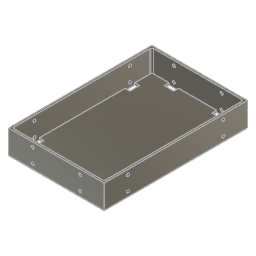
Arm Unit Bottom Case v1 (Autodesk Fusion 360 design; units mm, degrees)
Autodesk Fusion 360 part; units mm, degrees
sketch "Sketch1" plane through (0, 0, 0) normal (0, 0, 1) x (1, 0, 0) in component "case"
  line L0 (50, -75) -> (-50, -75)
  line L1 (-50, -75) -> (-50, 75)
  line L2 (-50, 75) -> (50, 75)
  line L3 (50, 75) -> (50, -75)
  line L4 (50, -75) -> (-50, 75) construction
  line L5 (-50, -75) -> (50, 75) construction
  dimension "d1" = 100
  dimension "d2" = 150
  constraint horizontal L0
  constraint perpendicular L0 L1
  constraint parallel L0 L2
  constraint parallel L1 L3
  constraint coincident L4 origin
  constraint coincident L5 origin
  measures "d1" distance of L1.end L2.end
  measures "d2" distance of L0.end L1.end
extrude "Extrude1" add sketch "Sketch1" along normal blind 25 in component "case"
sketch "Sketch1 (2)" plane through (0, 0, 25) normal (0, 0, 1) x (-1, 0, 0)
  line L0 (-50, -75) -> (50, -75)
  line L1 (50, -75) -> (50, 75)
  line L2 (50, 75) -> (-50, 75)
  line L3 (-50, 75) -> (-50, -75)
  line L4 (48, -73) -> (48, 73)
  line L5 (48, 73) -> (-48, 73)
  line L6 (-48, 73) -> (-48, -73)
  line L7 (-48, -73) -> (48, -73)
  dimension "d5" = -2
extrude "Extrude2" cut sketch "Sketch1 (2)" against normal blind 23 contours L4 L5 L6 L7 in component "case"
fillet "Fillet1" radius 2 4 edges at (48, -73, 13.5) (-48, -73, 13.5) (48, 73, 13.5) (-48, 73, 13.5) in component "case"
sketch "Sketch3" plane through (-50, 0, 0) normal (-1, 0, 0) x (0, -1, 0)
  line L0 (-75, 0) -> (75, 0)
  line L1 (75, 0) -> (75, 25)
  line L2 (75, 25) -> (-75, 25)
  line L3 (-75, 25) -> (-75, 0)
  circle A0 centre (-50, 20) radius 1.5
  dimension "d10" = 3
  measures "d10" diameter of A0
sketch "Sketch2" plane through (50, 0, 0) normal (1, 0, 0) x (0, 1, 0)
  line L0 (-75, 0) -> (75, 0)
  line L1 (75, 0) -> (75, 25)
  line L2 (75, 25) -> (-75, 25)
  line L3 (-75, 25) -> (-75, 0)
  circle A0 centre (-50, 20) radius 1.5
  dimension "d27" = 3
  measures "d27" diameter of A0
extrude "Extrude7" cut sketch "Sketch2" against normal blind 2 contours A0 in component "case"
extrude "Extrude3" cut sketch "Sketch3" against normal blind 2 contours A0 in component "case"
sketch "Sketch5" plane through (-50, 0, 0) normal (-1, 0, 0) x (0, -1, 0)
  circle A0 centre (-50, 20) radius 1.5
  line L0 (-75, 0) -> (75, 0)
  line L1 (75, 0) -> (75, 25)
  line L2 (75, 25) -> (-75, 25)
  line L3 (-75, 25) -> (-75, 0)
  circle A1 centre (-50, 5) radius 1.5
  dimension "d18" = 3
  measures "d18" diameter of A1
extrude "Extrude4" cut sketch "Sketch5" against normal blind 2 contours A1 in component "case"
sketch "Sketch6" plane through (-50, 0, 0) normal (-1, 0, 0) x (0, -1, 0)
  circle A0 centre (-50, 5) radius 1.5
  circle A1 centre (-50, 20) radius 1.5
  line L0 (-75, 0) -> (75, 0)
  line L1 (75, 0) -> (75, 25)
  line L2 (75, 25) -> (-75, 25)
  line L3 (-75, 25) -> (-75, 0)
  circle A2 centre (50, 5) radius 1.5
  dimension "d21" = 3
  measures "d21" diameter of A2
extrude "Extrude5" cut sketch "Sketch6" against normal blind 2 contours A2 in component "case"
sketch "Sketch7" plane through (-50, 0, 0) normal (-1, 0, 0) x (0, -1, 0)
  circle A0 centre (50, 5) radius 1.5
  circle A1 centre (-50, 5) radius 1.5
  circle A2 centre (-50, 20) radius 1.5
  line L0 (-75, 0) -> (75, 0)
  line L1 (75, 0) -> (75, 25)
  line L2 (75, 25) -> (-75, 25)
  line L3 (-75, 25) -> (-75, 0)
  circle A3 centre (50, 20) radius 1.5
  dimension "d24" = 3
  measures "d24" diameter of A3
extrude "Extrude6" cut sketch "Sketch7" against normal blind 2 contours A3 in component "case"
sketch "Sketch8" plane through (50, 0, 0) normal (1, 0, 0) x (0, 1, 0)
  circle A0 centre (-50, 20) radius 1.5
  line L0 (-75, 0) -> (75, 0)
  line L1 (75, 0) -> (75, 25)
  line L2 (75, 25) -> (-75, 25)
  line L3 (-75, 25) -> (-75, 0)
  circle A1 centre (-50, 5) radius 1.5
  dimension "d30" = 3
  measures "d30" diameter of A1
extrude "Extrude8" cut sketch "Sketch8" against normal blind 2 contours A1 in component "case"
sketch "Sketch9" plane through (50, 0, 0) normal (1, 0, 0) x (0, 1, 0)
  circle A0 centre (-50, 5) radius 1.5
  circle A1 centre (-50, 20) radius 1.5
  line L0 (-75, 0) -> (75, 0)
  line L1 (75, 0) -> (75, 25)
  line L2 (75, 25) -> (-75, 25)
  line L3 (-75, 25) -> (-75, 0)
  circle A2 centre (50, 20) radius 1.5
  dimension "d33" = 3
  measures "d33" diameter of A2
extrude "Extrude9" cut sketch "Sketch9" against normal blind 2 contours A2 in component "case"
sketch "Sketch10" plane through (50, 0, 0) normal (1, 0, 0) x (0, 1, 0)
  circle A0 centre (50, 20) radius 1.5
  circle A1 centre (-50, 5) radius 1.5
  circle A2 centre (-50, 20) radius 1.5
  line L0 (-75, 0) -> (75, 0)
  line L1 (75, 0) -> (75, 25)
  line L2 (75, 25) -> (-75, 25)
  line L3 (-75, 25) -> (-75, 0)
  circle A3 centre (50, 5) radius 1.5
  dimension "d36" = 3
  measures "d36" diameter of A3
extrude "Extrude10" cut sketch "Sketch10" against normal blind 2 contours A3 in component "case"
sketch "Sketch11" plane through (0, 75, 0) normal (0, 1, 0) x (-1, 0, 0)
  line L0 (-50, 0) -> (50, 0)
  line L1 (50, 0) -> (50, 25)
  line L2 (50, 25) -> (-50, 25)
  line L3 (-50, 25) -> (-50, 0)
  circle A0 centre (-25, 20) radius 1.5
  dimension "d39" = 3
  measures "d39" diameter of A0
extrude "Extrude11" cut sketch "Sketch11" against normal blind 2 contours A0 in component "case"
sketch "Sketch12" plane through (0, 75, 0) normal (0, 1, 0) x (-1, 0, 0)
  circle A0 centre (-25, 20) radius 1.5
  line L0 (-50, 0) -> (50, 0)
  line L1 (50, 0) -> (50, 25)
  line L2 (50, 25) -> (-50, 25)
  line L3 (-50, 25) -> (-50, 0)
  circle A1 centre (-25, 5) radius 1.5
  dimension "d42" = 3
  measures "d42" diameter of A1
extrude "Extrude12" cut sketch "Sketch12" against normal blind 2 contours A1 in component "case"
sketch "Sketch13" plane through (0, 75, 0) normal (0, 1, 0) x (-1, 0, 0)
  circle A0 centre (-25, 5) radius 1.5
  circle A1 centre (-25, 20) radius 1.5
  line L0 (-50, 0) -> (50, 0)
  line L1 (50, 0) -> (50, 25)
  line L2 (50, 25) -> (-50, 25)
  line L3 (-50, 25) -> (-50, 0)
  circle A2 centre (25, 5) radius 1.5
  dimension "d45" = 3
  measures "d45" diameter of A2
extrude "Extrude13" cut sketch "Sketch13" against normal blind 2 contours A2 in component "case"
sketch "Sketch14" plane through (0, 75, 0) normal (0, 1, 0) x (-1, 0, 0)
  circle A0 centre (25, 5) radius 1.5
  circle A1 centre (-25, 5) radius 1.5
  circle A2 centre (-25, 20) radius 1.5
  line L0 (-50, 0) -> (50, 0)
  line L1 (50, 0) -> (50, 25)
  line L2 (50, 25) -> (-50, 25)
  line L3 (-50, 25) -> (-50, 0)
  circle A3 centre (25, 20) radius 1.5
  dimension "d48" = 3
  measures "d48" diameter of A3
extrude "Extrude14" cut sketch "Sketch14" against normal blind 2 contours A3 in component "case"
sketch "Sketch15" plane through (0, -75, 0) normal (0, -1, 0) x (1, 0, 0)
  line L0 (-50, 0) -> (50, 0)
  line L1 (50, 0) -> (50, 25)
  line L2 (50, 25) -> (-50, 25)
  line L3 (-50, 25) -> (-50, 0)
  circle A0 centre (-25, 20) radius 1.5
  dimension "d51" = 3
  measures "d51" diameter of A0
extrude "Extrude15" cut sketch "Sketch15" against normal blind 2 contours A0 in component "case"
sketch "Sketch16" plane through (0, -75, 0) normal (0, -1, 0) x (1, 0, 0)
  circle A0 centre (-25, 20) radius 1.5
  line L0 (-50, 0) -> (50, 0)
  line L1 (50, 0) -> (50, 25)
  line L2 (50, 25) -> (-50, 25)
  line L3 (-50, 25) -> (-50, 0)
  circle A1 centre (-25, 5) radius 1.5
  dimension "d54" = 3
  measures "d54" diameter of A1
extrude "Extrude16" cut sketch "Sketch16" against normal blind 2 contours A1 in component "case"
sketch "Sketch17" plane through (0, -75, 0) normal (0, -1, 0) x (1, 0, 0)
  circle A0 centre (-25, 5) radius 1.5
  circle A1 centre (-25, 20) radius 1.5
  line L0 (-50, 0) -> (50, 0)
  line L1 (50, 0) -> (50, 25)
  line L2 (50, 25) -> (-50, 25)
  line L3 (-50, 25) -> (-50, 0)
  circle A2 centre (25, 5) radius 1.5
  dimension "d57" = 3
  measures "d57" diameter of A2
extrude "Extrude17" cut sketch "Sketch17" against normal blind 2 contours A2 in component "case"
sketch "Sketch18" plane through (0, -75, 0) normal (0, -1, 0) x (1, 0, 0)
  circle A0 centre (25, 5) radius 1.5
  circle A1 centre (-25, 5) radius 1.5
  circle A2 centre (-25, 20) radius 1.5
  line L0 (-50, 0) -> (50, 0)
  line L1 (50, 0) -> (50, 25)
  line L2 (50, 25) -> (-50, 25)
  line L3 (-50, 25) -> (-50, 0)
  circle A3 centre (25, 20) radius 1.5
  dimension "d60" = 3
  measures "d60" diameter of A3
extrude "Extrude18" cut sketch "Sketch18" against normal blind 2 contours A3 in component "case"
sketch "Sketch20" plane through (0, 0, 2) normal (0, 0, 1) x (-1, 0, 0)
  arc A0 (46, -73) -> (48, -71) centre (46, -71) ccw
  line L0 (48, -71) -> (48, 71)
  arc A1 (48, 71) -> (46, 73) centre (46, 71) ccw
  line L1 (46, 73) -> (-46, 73)
  arc A2 (-46, 73) -> (-48, 71) centre (-46, 71) ccw
  line L2 (-48, 71) -> (-48, -71)
  arc A3 (-48, -71) -> (-46, -73) centre (-46, -71) ccw
  line L3 (-46, -73) -> (46, -73)
  line L4 (-48, -45) -> (-43, -45)
  line L5 (-43, -45) -> (-43, -55)
  line L6 (-43, -55) -> (-48, -55)
  line L7 (-48, -55) -> (-48, -45)
  dimension "d65" = 5
  dimension "d66" = 10
  constraint horizontal L4
  constraint vertical L5
  constraint horizontal L6
  constraint vertical L7
  measures "d65" distance of L4.start L4.end
  measures "d66" distance of L4.start L6.end
extrude "Extrude19" cut sketch "Sketch20" against normal blind 2 contours L2 L4 L5 L6 L7 in component "case"
sketch "Sketch21" plane through (0, 0, 2) normal (0, 0, 1) x (-1, 0, 0)
  line L0 (-43, -55) -> (-48, -55)
  line L1 (-48, -55) -> (-48, -71)
  arc A0 (-48, -71) -> (-46, -73) centre (-46, -71) ccw
  line L2 (-46, -73) -> (46, -73)
  arc A1 (46, -73) -> (48, -71) centre (46, -71) ccw
  line L3 (48, -71) -> (48, 71)
  arc A2 (48, 71) -> (46, 73) centre (46, 71) ccw
  line L4 (46, 73) -> (-46, 73)
  arc A3 (-46, 73) -> (-48, 71) centre (-46, 71) ccw
  line L5 (-48, 71) -> (-48, -45)
  line L6 (-48, -45) -> (-43, -45)
  line L7 (-43, -45) -> (-43, -55)
  line L8 (-20, -73) -> (-30, -73)
  line L9 (-30, -73) -> (-30, -68)
  line L10 (-30, -68) -> (-20, -68)
  line L11 (-20, -68) -> (-20, -73)
  dimension "d69" = 10
  dimension "d70" = 5
  constraint horizontal L8
  constraint vertical L9
  constraint horizontal L10
  constraint vertical L11
  measures "d69" distance of L8.start L8.end
  measures "d70" distance of L8.start L10.end
extrude "Extrude20" cut sketch "Sketch21" against normal blind 2 contours L2 L8 L9 L10 L11 in component "case"
sketch "Sketch22" plane through (0, 0, 2) normal (0, 0, 1) x (-1, 0, 0)
  line L0 (-20, -68) -> (-20, -73)
  line L1 (-20, -73) -> (46, -73)
  arc A0 (46, -73) -> (48, -71) centre (46, -71) ccw
  line L2 (48, -71) -> (48, 71)
  arc A1 (48, 71) -> (46, 73) centre (46, 71) ccw
  line L3 (46, 73) -> (-46, 73)
  arc A2 (-46, 73) -> (-48, 71) centre (-46, 71) ccw
  line L4 (-48, 71) -> (-48, -45)
  line L5 (-48, -45) -> (-43, -45)
  line L6 (-43, -45) -> (-43, -55)
  line L7 (-43, -55) -> (-48, -55)
  line L8 (-48, -55) -> (-48, -71)
  arc A3 (-48, -71) -> (-46, -73) centre (-46, -71) ccw
  line L9 (-46, -73) -> (-30, -73)
  line L10 (-30, -73) -> (-30, -68)
  line L11 (-30, -68) -> (-20, -68)
  line L12 (30, -73) -> (20, -73)
  line L13 (20, -73) -> (20, -68)
  line L14 (20, -68) -> (30, -68)
  line L15 (30, -68) -> (30, -73)
  dimension "d73" = 10
  dimension "d74" = 5
  constraint horizontal L12
  constraint vertical L13
  constraint horizontal L14
  constraint vertical L15
  measures "d73" distance of L12.start L12.end
  measures "d74" distance of L12.start L14.end
extrude "Extrude21" cut sketch "Sketch22" against normal blind 2 contours L1 L12 L13 L14 L15 in component "case"
sketch "Sketch23" plane through (0, 0, 2) normal (0, 0, 1) x (-1, 0, 0)
  line L0 (30, -68) -> (30, -73)
  line L1 (30, -73) -> (46, -73)
  arc A0 (46, -73) -> (48, -71) centre (46, -71) ccw
  line L2 (48, -71) -> (48, 71)
  arc A1 (48, 71) -> (46, 73) centre (46, 71) ccw
  line L3 (46, 73) -> (-46, 73)
  arc A2 (-46, 73) -> (-48, 71) centre (-46, 71) ccw
  line L4 (-48, 71) -> (-48, -45)
  line L5 (-48, -45) -> (-43, -45)
  line L6 (-43, -45) -> (-43, -55)
  line L7 (-43, -55) -> (-48, -55)
  line L8 (-48, -55) -> (-48, -71)
  arc A3 (-48, -71) -> (-46, -73) centre (-46, -71) ccw
  line L9 (-46, -73) -> (-30, -73)
  line L10 (-30, -73) -> (-30, -68)
  line L11 (-30, -68) -> (-20, -68)
  line L12 (-20, -68) -> (-20, -73)
  line L13 (-20, -73) -> (20, -73)
  line L14 (20, -73) -> (20, -68)
  line L15 (20, -68) -> (30, -68)
  line L16 (48, -45) -> (43, -45)
  line L17 (43, -45) -> (43, -55)
  line L18 (43, -55) -> (48, -55)
  line L19 (48, -55) -> (48, -45)
  dimension "d77" = 5
  dimension "d78" = 10
  constraint horizontal L16
  constraint vertical L17
  constraint horizontal L18
  constraint vertical L19
  measures "d77" distance of L16.start L16.end
  measures "d78" distance of L16.start L18.end
extrude "Extrude22" cut sketch "Sketch23" against normal blind 2 contours L2 L16 L17 L18 L19 in component "case"
sketch "Sketch24" plane through (0, 0, 2) normal (0, 0, 1) x (-1, 0, 0)
  line L0 (48, -55) -> (43, -55)
  line L1 (43, -55) -> (43, -45)
  line L2 (43, -45) -> (48, -45)
  line L3 (48, -45) -> (48, 71)
  arc A0 (48, 71) -> (46, 73) centre (46, 71) ccw
  line L4 (46, 73) -> (-46, 73)
  arc A1 (-46, 73) -> (-48, 71) centre (-46, 71) ccw
  line L5 (-48, 71) -> (-48, -45)
  line L6 (-48, -45) -> (-43, -45)
  line L7 (-43, -45) -> (-43, -55)
  line L8 (-43, -55) -> (-48, -55)
  line L9 (-48, -55) -> (-48, -71)
  arc A2 (-48, -71) -> (-46, -73) centre (-46, -71) ccw
  line L10 (-46, -73) -> (-30, -73)
  line L11 (-30, -73) -> (-30, -68)
  line L12 (-30, -68) -> (-20, -68)
  line L13 (-20, -68) -> (-20, -73)
  line L14 (-20, -73) -> (20, -73)
  line L15 (20, -73) -> (20, -68)
  line L16 (20, -68) -> (30, -68)
  line L17 (30, -68) -> (30, -73)
  line L18 (30, -73) -> (46, -73)
  arc A3 (46, -73) -> (48, -71) centre (46, -71) ccw
  line L19 (48, -71) -> (48, -55)
  line L20 (-48, 45) -> (-43, 45)
  line L21 (-43, 45) -> (-43, 55)
  line L22 (-43, 55) -> (-48, 55)
  line L23 (-48, 55) -> (-48, 45)
  dimension "d81" = 5
  dimension "d82" = 10
  constraint horizontal L20
  constraint vertical L21
  constraint horizontal L22
  constraint vertical L23
  measures "d81" distance of L20.start L20.end
  measures "d82" distance of L20.start L22.end
extrude "Extrude23" cut sketch "Sketch24" against normal blind 2 contours L5 L20 L21 L22 L23 in component "case"
sketch "Sketch25" plane through (0, 0, 2) normal (0, 0, 1) x (-1, 0, 0)
  line L0 (-48, 55) -> (-43, 55)
  line L1 (-43, 55) -> (-43, 45)
  line L2 (-43, 45) -> (-48, 45)
  line L3 (-48, 45) -> (-48, -45)
  line L4 (-48, -45) -> (-43, -45)
  line L5 (-43, -45) -> (-43, -55)
  line L6 (-43, -55) -> (-48, -55)
  line L7 (-48, -55) -> (-48, -71)
  arc A0 (-48, -71) -> (-46, -73) centre (-46, -71) ccw
  line L8 (-46, -73) -> (-30, -73)
  line L9 (-30, -73) -> (-30, -68)
  line L10 (-30, -68) -> (-20, -68)
  line L11 (-20, -68) -> (-20, -73)
  line L12 (-20, -73) -> (20, -73)
  line L13 (20, -73) -> (20, -68)
  line L14 (20, -68) -> (30, -68)
  line L15 (30, -68) -> (30, -73)
  line L16 (30, -73) -> (46, -73)
  arc A1 (46, -73) -> (48, -71) centre (46, -71) ccw
  line L17 (48, -71) -> (48, -55)
  line L18 (48, -55) -> (43, -55)
  line L19 (43, -55) -> (43, -45)
  line L20 (43, -45) -> (48, -45)
  line L21 (48, -45) -> (48, 71)
  arc A2 (48, 71) -> (46, 73) centre (46, 71) ccw
  line L22 (46, 73) -> (-46, 73)
  arc A3 (-46, 73) -> (-48, 71) centre (-46, 71) ccw
  line L23 (-48, 71) -> (-48, 55)
  line L24 (-20, 68) -> (-30, 68)
  line L25 (-30, 68) -> (-30, 73)
  line L26 (-30, 73) -> (-20, 73)
  line L27 (-20, 73) -> (-20, 68)
  dimension "d85" = 10
  dimension "d86" = 5
  constraint horizontal L24
  constraint vertical L25
  constraint horizontal L26
  constraint vertical L27
  measures "d85" distance of L24.start L24.end
  measures "d86" distance of L24.start L26.end
extrude "Extrude24" cut sketch "Sketch25" against normal blind 2 contours L22 L24 L25 L26 L27 in component "case"
sketch "Sketch26" plane through (0, 0, 2) normal (0, 0, 1) x (-1, 0, 0)
  line L0 (-20, 73) -> (-20, 68)
  line L1 (-20, 68) -> (-30, 68)
  line L2 (-30, 68) -> (-30, 73)
  line L3 (-30, 73) -> (-46, 73)
  arc A0 (-46, 73) -> (-48, 71) centre (-46, 71) ccw
  line L4 (-48, 71) -> (-48, 55)
  line L5 (-48, 55) -> (-43, 55)
  line L6 (-43, 55) -> (-43, 45)
  line L7 (-43, 45) -> (-48, 45)
  line L8 (-48, 45) -> (-48, -45)
  line L9 (-48, -45) -> (-43, -45)
  line L10 (-43, -45) -> (-43, -55)
  line L11 (-43, -55) -> (-48, -55)
  line L12 (-48, -55) -> (-48, -71)
  arc A1 (-48, -71) -> (-46, -73) centre (-46, -71) ccw
  line L13 (-46, -73) -> (-30, -73)
  line L14 (-30, -73) -> (-30, -68)
  line L15 (-30, -68) -> (-20, -68)
  line L16 (-20, -68) -> (-20, -73)
  line L17 (-20, -73) -> (20, -73)
  line L18 (20, -73) -> (20, -68)
  line L19 (20, -68) -> (30, -68)
  line L20 (30, -68) -> (30, -73)
  line L21 (30, -73) -> (46, -73)
  arc A2 (46, -73) -> (48, -71) centre (46, -71) ccw
  line L22 (48, -71) -> (48, -55)
  line L23 (48, -55) -> (43, -55)
  line L24 (43, -55) -> (43, -45)
  line L25 (43, -45) -> (48, -45)
  line L26 (48, -45) -> (48, 71)
  arc A3 (48, 71) -> (46, 73) centre (46, 71) ccw
  line L27 (46, 73) -> (-20, 73)
  line L28 (20, 73) -> (30, 73)
  line L29 (30, 73) -> (30, 68)
  line L30 (30, 68) -> (20, 68)
  line L31 (20, 68) -> (20, 73)
  dimension "d89" = 10
  dimension "d90" = 5
  constraint horizontal L28
  constraint vertical L29
  constraint horizontal L30
  constraint vertical L31
  measures "d89" distance of L28.start L28.end
  measures "d90" distance of L28.start L30.end
extrude "Extrude25" cut sketch "Sketch26" against normal blind 2 contours L27 L28 L29 L30 L31 in component "case"
sketch "Sketch27" plane through (0, 0, 2) normal (0, 0, 1) x (-1, 0, 0)
  line L0 (20, 68) -> (20, 73)
  line L1 (20, 73) -> (-20, 73)
  line L2 (-20, 73) -> (-20, 68)
  line L3 (-20, 68) -> (-30, 68)
  line L4 (-30, 68) -> (-30, 73)
  line L5 (-30, 73) -> (-46, 73)
  arc A0 (-46, 73) -> (-48, 71) centre (-46, 71) ccw
  line L6 (-48, 71) -> (-48, 55)
  line L7 (-48, 55) -> (-43, 55)
  line L8 (-43, 55) -> (-43, 45)
  line L9 (-43, 45) -> (-48, 45)
  line L10 (-48, 45) -> (-48, -45)
  line L11 (-48, -45) -> (-43, -45)
  line L12 (-43, -45) -> (-43, -55)
  line L13 (-43, -55) -> (-48, -55)
  line L14 (-48, -55) -> (-48, -71)
  arc A1 (-48, -71) -> (-46, -73) centre (-46, -71) ccw
  line L15 (-46, -73) -> (-30, -73)
  line L16 (-30, -73) -> (-30, -68)
  line L17 (-30, -68) -> (-20, -68)
  line L18 (-20, -68) -> (-20, -73)
  line L19 (-20, -73) -> (20, -73)
  line L20 (20, -73) -> (20, -68)
  line L21 (20, -68) -> (30, -68)
  line L22 (30, -68) -> (30, -73)
  line L23 (30, -73) -> (46, -73)
  arc A2 (46, -73) -> (48, -71) centre (46, -71) ccw
  line L24 (48, -71) -> (48, -55)
  line L25 (48, -55) -> (43, -55)
  line L26 (43, -55) -> (43, -45)
  line L27 (43, -45) -> (48, -45)
  line L28 (48, -45) -> (48, 71)
  arc A3 (48, 71) -> (46, 73) centre (46, 71) ccw
  line L29 (46, 73) -> (30, 73)
  line L30 (30, 73) -> (30, 68)
  line L31 (30, 68) -> (20, 68)
  line L32 (48, 45) -> (43, 45)
  line L33 (43, 45) -> (43, 55)
  line L34 (43, 55) -> (48, 55)
  line L35 (48, 55) -> (48, 45)
  dimension "d93" = 5
  dimension "d94" = 10
  constraint horizontal L32
  constraint vertical L33
  constraint horizontal L34
  constraint vertical L35
  measures "d93" distance of L32.start L32.end
  measures "d94" distance of L32.start L34.end
extrude "Extrude26" cut sketch "Sketch27" against normal blind 2 contours L28 L32 L33 L34 L35 in component "case"
sketch "Sketch28" plane through (0, 0, 2) normal (0, 0, 1) x (-1, 0, 0)
  line L0 (43, 55) -> (48, 55)
  line L1 (48, 55) -> (48, 71)
  arc A0 (48, 71) -> (46, 73) centre (46, 71) ccw
  line L2 (46, 73) -> (30, 73)
  line L3 (30, 73) -> (30, 68)
  line L4 (30, 68) -> (20, 68)
  line L5 (20, 68) -> (20, 73)
  line L6 (20, 73) -> (-20, 73)
  line L7 (-20, 73) -> (-20, 68)
  line L8 (-20, 68) -> (-30, 68)
  line L9 (-30, 68) -> (-30, 73)
  line L10 (-30, 73) -> (-46, 73)
  arc A1 (-46, 73) -> (-48, 71) centre (-46, 71) ccw
  line L11 (-48, 71) -> (-48, 55)
  line L12 (-48, 55) -> (-43, 55)
  line L13 (-43, 55) -> (-43, 45)
  line L14 (-43, 45) -> (-48, 45)
  line L15 (-48, 45) -> (-48, -45)
  line L16 (-48, -45) -> (-43, -45)
  line L17 (-43, -45) -> (-43, -55)
  line L18 (-43, -55) -> (-48, -55)
  line L19 (-48, -55) -> (-48, -71)
  arc A2 (-48, -71) -> (-46, -73) centre (-46, -71) ccw
  line L20 (-46, -73) -> (-30, -73)
  line L21 (-30, -73) -> (-30, -68)
  line L22 (-30, -68) -> (-20, -68)
  line L23 (-20, -68) -> (-20, -73)
  line L24 (-20, -73) -> (20, -73)
  line L25 (20, -73) -> (20, -68)
  line L26 (20, -68) -> (30, -68)
  line L27 (30, -68) -> (30, -73)
  line L28 (30, -73) -> (46, -73)
  arc A3 (46, -73) -> (48, -71) centre (46, -71) ccw
  line L29 (48, -71) -> (48, -55)
  line L30 (48, -55) -> (43, -55)
  line L31 (43, -55) -> (43, -45)
  line L32 (43, -45) -> (48, -45)
  line L33 (48, -45) -> (48, 45)
  line L34 (48, 45) -> (43, 45)
  line L35 (43, 45) -> (43, 55)
  line L36 (-10.0989, -28.0489, -5) -> (-10.0989, 11.9511, -5) construction
  line L37 (-10.0989, 11.9511, -5) -> (4.9011, 11.9511, -5) construction
  line L38 (4.9011, 11.9511, -5) -> (4.9011, -28.0489, -5) construction
  line L39 (4.9011, -28.0489, -5) -> (-10.0989, -28.0489, -5) construction
  dimension "d97" = 10
  text T0 "Prototype" font "Arial" height 10 align left top in box 40 x 15 at (-10.0989, -28.0489) x (0, 1) y (1, 0) spacing 1
emboss "Emboss1" depth -0.25 profiles "Sketch28" section 1 text T0 onto face at (-14.3333, 15, 0) in component "case"
component "case" placed x (1, 0, 0) y (0, 1, 0) z (0, 0, 1) at (0, 0, 0)
